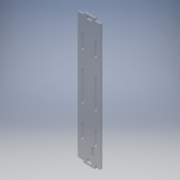
# Autodesk Inventor part: Right_wall
Saved by Autodesk Inventor 2016 (Build 200138000, 138)
## iProperties
Created: 2015-06-19
Part Number: Right_wall
Material: Generic
Document SubType Name: Modeling
Designer: Openlab
Density: 1 g/cm^3
Appearance: Polycarbonate - Clear
Author: Openlab
Autodesk Inventor part; units mm, degrees
ref_plane "YZ Plane" through (0, 0, 0) normal (1, 0, 0) x (0, 1, 0)
ref_plane "XZ Plane" through (0, 0, 0) normal (0, 1, 0) x (-1, 0, 0)
ref_plane "XY Plane" through (0, 0, 0) normal (0, 0, 1) x (1, 0, 0)
sketch "Sketch1" plane through (0, 0, 0) normal (0, 1, 0) x (-1, 0, 0)
  line L0 (26.5, -25) -> (23.5, -25)
  line L1 (26.5, -43) -> (23.5, -43)
  line L2 (26.5, -68) -> (23.5, -68)
  line L3 (26.5, -108) -> (23.5, -108)
  line L4 (8, -68) -> (5, -68)
  line L5 (8, -108) -> (5, -108)
  line L6 (8, -43) -> (5, -43)
  line L7 (8, -25) -> (5, -25)
  line L8 (23.5, -108) -> (23.5, -68)
  line L9 (23.5, -43) -> (23.5, -25)
  line L10 (8, -108) -> (8, -68)
  line L11 (8, -43) -> (8, -25)
  line L12 (15.75, -68) -> (15.75, -97) construction
  line L13 (23.5, -133) -> (23.5, -151)
  line L14 (23.5, -151) -> (26.5, -151)
  line L15 (5, -151) -> (8, -151)
  line L16 (8, -133) -> (8, -151)
  line L17 (26.5, -133) -> (23.5, -133)
  line L18 (8, -133) -> (5, -133)
  line L19 (12.8, -156) -> (11, -156)
  line L20 (11, -156) -> (11, -166)
  line L21 (11, -166) -> (12.8, -166)
  line L22 (12.8, -166) -> (12.8, -156)
  line L23 (23.5, 0) -> (23.5, 3)
  line L24 (23.5, 3) -> (8, 3)
  line L25 (8, 3) -> (8, 0)
  line L26 (8, 0) -> (0, 0)
  line L27 (23.5, -176) -> (23.5, -179)
  line L28 (23.5, -179) -> (8, -179)
  line L29 (8, -179) -> (8, -176)
  line L30 (8, -176) -> (0, -176)
  line L31 (19.25, 0) -> (12.25, 0)
  line L32 (12.25, 0) -> (12.25, -3)
  line L33 (12.25, -3) -> (19.25, -3)
  line L34 (19.25, -3) -> (19.25, 0)
  line L35 (19.25, -173) -> (12.25, -173)
  line L36 (12.25, -173) -> (12.25, -176)
  line L37 (12.25, -176) -> (19.25, -176)
  line L38 (19.25, -176) -> (19.25, -173)
  line L39 (26.5, -25) -> (26.5, -43)
  line L40 (26.5, -68) -> (26.5, -108)
  line L41 (26.5, -133) -> (26.5, -151)
  line L42 (5, -151) -> (5, -133)
  line L43 (5, -108) -> (5, -68)
  line L44 (5, -43) -> (5, -25)
  line L45 (31.5, 0) -> (31.5, -176)
  line L46 (31.5, -176) -> (23.5, -176)
  line L47 (0, -176) -> (0, 0)
  line L48 (31.5, 0) -> (23.5, 0)
  dimension "d7" = 18
  dimension "d8" = 25
  dimension "d9" = 40
  dimension "d45" = 18
  dimension "d49" = 1.8
  dimension "d51" = 10
  dimension "d53" = 3
  dimension "d56" = 10
  dimension "d57" = 7
  dimension "d58" = 3
  dimension "d59" = 3
  dimension "d64" = 25
  dimension "d66" = 25
  dimension "d67" = 25
  dimension "d68" = 15.5
  dimension "d69" = 5
  constraints: 98 end point, 18 collinear, 12 perpendicular, 10 equal length, 9 parallel, 5 vertical, 4 horizontal, 3 point on line, 2 coincident, 8 other
  measures "d7" distance between parallel lines of L1 L0
  measures "d8" distance between parallel lines of L2 L1
  measures "d9" distance between parallel lines of L3 L2
  measures "d45" distance of L13.start L13.end
  measures "d49" distance of L19.start L19.end
  measures "d51" distance of L21.end L19.start
  measures "d53" distance between parallel lines of L16 L20
  measures "d56" distance between parallel lines of L30 L21
  measures "d57" distance of L32.end L33.end
  measures "d58" distance of L31.end L32.end
  measures "d59" distance of L0.start L0.end
  measures "d64" distance between parallel lines of L0 L48
  measures "d66" distance between parallel lines of L46 L14
  measures "d67" distance between parallel lines of L3 L17
  measures "d68" distance between parallel lines of L10 L8
  measures "d69" distance between parallel lines of L47 L43
extrude "Extrusion3" add sketch "Sketch1" along normal blind 3
body "Solid3"
